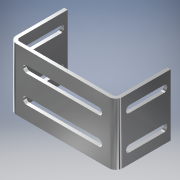
# Autodesk Inventor part: trackball_cup
Saved by Autodesk Inventor 2018 (Build 220112000, 112)
## iProperties
Created: 2018-04-06
Part Number: trackball_cup
Material: アルミニウム 6061
Document SubType Name: Sheet Metal
Designer: NaMACHAN
Density: 2.7 g/cm^3
Sheet Metal Rule: Default_mm
Appearance: アルミニウム - フラット
Flat Pattern Width: 3.59 cm
Flat Pattern Length: 11.9048 cm
Flat Pattern Area: 42.7382 cm^2
Sheet Metal Width: 35.900 mm
Sheet Metal Length: 119.048 mm
Sheet Metal Area: 4273.816 mm^2
Author: NaMACHAN
Autodesk Inventor part; units mm, degrees
ref_plane "YZ Plane" through (0, 0, 0) normal (1, 0, 0) x (0, 1, 0)
ref_plane "XZ Plane" through (0, 0, 0) normal (0, 1, 0) x (-1, 0, 0)
ref_plane "XY Plane" through (0, 0, 0) normal (0, 0, 1) x (1, 0, 0)
sketch "スケッチ1" plane through (0, 0, 0) normal (0, 1, 0) x (-1, 0, 0)
  line L0 (-29, -17.95) -> (29, -17.95)
  line L1 (29, -17.95) -> (29, 17.95)
  line L2 (29, 17.95) -> (-29, 17.95)
  line L3 (-29, 17.95) -> (-29, -17.95)
  line L4 (-29, -17.95) -> (29, 17.95) construction
  line L5 (29, -17.95) -> (-29, 17.95) construction
  point P0 (0, 0)
  dimension "d0" = 35.9
  dimension "d1" = 58
  measures "d0" distance of L0.end L1.end
  measures "d1" distance of L0.start L0.end
extrude "プレート1" add sketch "スケッチ1" along normal blind 2
sketch "スケッチ2" plane through (29, 0, 17.95) normal (1, 0, 0) x (0, 0, -1)
  line L0 (0, 2) -> (35.9, 2)
  line L1 (35.9, 2) -> (0, 2)
  line L2 (0, 2) -> (0, 32)
  line L3 (0, 32) -> (35.9, 32)
  line L4 (35.9, 32) -> (35.9, 2)
  point P0 (17.95, 0)
  dimension "d3" = 30
  measures "d3" distance of L3.end L0.end
sheet face with bend "面2" sketch "スケッチ2" thickness 2 toward (1, 0, 0) bend radius 2
bend "曲げ1"
sketch "スケッチ3" plane through (-29, 0, -17.95) normal (-1, 0, 0) x (0, 0, 1)
  line L0 (0, 0) -> (0, 2)
  line L1 (0, 32) -> (35.9, 32)
  line L2 (0, 2) -> (35.9, 2)
  line L3 (35.9, 2) -> (35.9, 32)
  line L4 (35.9, 32) -> (0, 32)
  line L5 (0, 32) -> (0, 2)
  point P0 (17.95, 0)
sheet face with bend "面3" sketch "スケッチ3" thickness 2 toward (-1, 0, 0) bend radius 2
bend "曲げ2"
sketch "スケッチ4" plane through (-31, 0, -17.95) normal (-1, 0, 0) x (0, 0, 1)
  line L0 (6, 28) -> (6, 8)
  arc A0 (6, 8) -> (10, 8) centre (8, 8) ccw
  line L1 (10, 8) -> (10, 28)
  arc A1 (10, 28) -> (6, 28) centre (8, 28) ccw
  line L2 (0, 32) -> (35.9, 32) projected
  line L3 (35.9, 4) -> (0, 4) projected
  line L4 (0, 4) -> (0, 32) projected
  line L5 (25.9, 28) -> (25.9, 8)
  arc A2 (25.9, 8) -> (29.9, 8) centre (27.9, 8) ccw
  line L6 (29.9, 8) -> (29.9, 28)
  arc A3 (29.9, 28) -> (25.9, 28) centre (27.9, 28) ccw
  line L7 (35.9, 32) -> (35.9, 4) projected
  point P0 (17.95, 0)
  dimension "d14" = 2
  dimension "d15" = 4
  dimension "d16" = 4
  dimension "d17" = 6
  dimension "d18" = 2
  dimension "d19" = 6
  constraints: 8 end point, 8 point on circle, 8 tangent, 4 centre point, 2 horizontal alignment, 2 parallel, 2 vertical
  measures "d14" radius of A1
  measures "d15" distance from line of L2 A1.centre
  measures "d16" distance from line of L3 A0.centre
  measures "d17" distance between parallel lines of L4 L0
  measures "d18" radius of A3
  measures "d19" distance between parallel lines of L7 L6
extrude "押し出し1" cut sketch "スケッチ4" against normal blind 100 contours A1 L1 A0 L0 | A3 L6 A2 L5
sketch "スケッチ5" plane through (0, 2, 0) normal (0, 1, 0) x (1, 0, 0)
  line L0 (-21, -9.95) -> (21, -9.95)
  arc A0 (21, -9.95) -> (21, -5.95) centre (21, -7.95) ccw
  line L1 (21, -5.95) -> (-21, -5.95)
  arc A1 (-21, -5.95) -> (-21, -9.95) centre (-21, -7.95) ccw
  line L2 (-21, 5.95) -> (21, 5.95)
  arc A2 (21, 5.95) -> (21, 9.95) centre (21, 7.95) ccw
  line L3 (21, 9.95) -> (-21, 9.95)
  arc A3 (-21, 9.95) -> (-21, 5.95) centre (-21, 7.95) ccw
  line L4 (-27, 17.95) -> (27, 17.95) projected
  line L5 (27, -17.95) -> (-27, -17.95) projected
  line L6 (-27, 17.95) -> (-27, -17.95) projected
  line L7 (27, -17.95) -> (27, 17.95) projected
  point P0 (0, 0)
  dimension "d22" = 2
  dimension "d23" = 2
  dimension "d25" = 10
  dimension "d26" = 10
  dimension "d27" = 6
  dimension "d28" = 6
  dimension "d29" = 6
  dimension "d30" = 6
  constraints: 8 end point, 8 point on circle, 8 tangent, 4 centre point, 2 horizontal, 2 parallel
  measures "d22" radius of A1
  measures "d23" radius of A3
  measures "d25" distance from line of L4 A3.centre
  measures "d26" distance from line of L5 A1.centre
  measures "d27" distance from line of L6 A1.centre
  measures "d28" distance from line of L6 A3.centre
  measures "d29" distance from line of L7 A2.centre
  measures "d30" distance from line of L7 A0.centre
extrude "押し出し2" cut sketch "スケッチ5" against normal blind 3 contours A1 L1 A0 L0 | A3 L3 A2 L2
equation "\"d2\" = Thickness"
equation "\"d4\" = BendRadius"
equation "\"d5\" = BendReliefWidth"
equation "\"d7\" = MinimumRemnant"
equation "\"d6\" = BendReliefDepth"
equation "\"d8\" = TransitionRadius"
equation "\"d9\" = BendRadius"
equation "\"d10\" = BendReliefWidth"
equation "\"d12\" = MinimumRemnant"
equation "\"d11\" = BendReliefDepth"
equation "\"d13\" = TransitionRadius"
equation "\"BendRadius\" = Thickness"
equation "\"BendReliefWidth\" = Thickness"
equation "\"BendReliefDepth\" = 0.5 * Thickness"
equation "\"CornerReliefSize\" = 4 * Thickness"
equation "\"MinimumRemnant\" = 2 * Thickness"
equation "\"TransitionRadius\" = BendRadius"
equation "\"JacobiRadiusSize\" = BendRadius"
equation "\"GapSize\" = Thickness"
equation "\"Thickness\" = 2"
